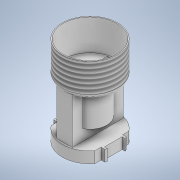
# Autodesk Inventor part: bulbholder
Saved by Autodesk Inventor 2020 (Build 240168000, 168)
## iProperties
Created: 2020-09-10
Part Number: bulbholder
Material: Generic
Document SubType Name: Modeling
Designer: zgoh017
Density: 1 g/cm^3
Appearance: Default
Author: zgoh017
Autodesk Inventor part; units mm, degrees
ref_plane "YZ Plane" through (0, 0, 0) normal (1, 0, 0) x (0, 1, 0)
ref_plane "XZ Plane" through (0, 0, 0) normal (0, 1, 0) x (-1, 0, 0)
ref_plane "XY Plane" through (0, 0, 0) normal (0, 0, 1) x (1, 0, 0)
sketch "Sketch1" plane through (0, 0, 0) normal (0, 1, 0) x (-1, 0, 0)
  circle A0 centre (0, 0) radius 12.5
  dimension "d0" = 25
  constraints: 1 centre point, 1 coincident
  measures "d0" diameter of A0
extrude "Extrusion1" add sketch "Sketch1" along normal blind 5
sketch "Sketch2" plane through (0, 5, 0) normal (0, 1, 0) x (1, 0, 0)
  circle A0 centre (0, 0) radius 12.5 projected
  line L0 (-12.5, 0) -> (-10.5, 0)
  line L1 (-10.5, 0) -> (-10.5, 4)
  line L2 (-10.5, 4) -> (-11.8427, 4)
  line L3 (-10.5, 0) -> (-10.5, -4)
  line L4 (-10.5, -4) -> (-11.8427, -4)
  line L5 (12.5, 0) -> (10.5, 0)
  line L6 (10.5, 0) -> (10.5, 4)
  line L7 (10.5, 4) -> (11.8427, 4)
  line L8 (10.5, 0) -> (10.5, -4)
  line L9 (10.5, -4) -> (11.8427, -4)
  dimension "d3" = 2
  dimension "d4" = 4
  dimension "d5" = 4
  dimension "d6" = 2
  dimension "d28" = 4
  dimension "d29" = 4
  constraints: 20 end point, 6 point on circle, 5 perpendicular, 3 horizontal, 2 point on line
  measures "d3" distance of L0.start L0.end
  measures "d4" distance of L0.end L1.end
  measures "d5" distance of L0.end L3.end
  measures "d6" distance of L5.start L5.end
  measures "d28" distance of L5.end L6.end
  measures "d29" distance of L5.end L8.end
extrude "Extrusion2" cut sketch "Sketch2" against normal through all contours L5 L6 L7 A0 | A0 L9 L8 L5 | L2 L1 L0 A0 | A0 L0 L3 L4
sketch "Sketch4" plane through (0, 5, 0) normal (0, 1, 0) x (1, 0, 0)
  line L0 (3.5, -11.5) -> (-3.5, -11.5)
  line L1 (-3.5, -11.5) -> (-3.5, 11.5)
  line L2 (-3.5, 11.5) -> (3.5, 11.5)
  line L3 (3.5, 11.5) -> (3.5, -11.5)
  line L4 (3.5, -11.5) -> (-3.5, 11.5) construction
  line L5 (-3.5, -11.5) -> (3.5, 11.5) construction
  point P0 (0, 0)
  dimension "d9" = 7
  dimension "d10" = 23
  constraints: 12 end point, 2 midpoint, 2 parallel, 1 horizontal, 1 perpendicular
  measures "d9" distance of L1.end L2.end
  measures "d10" distance of L0.end L1.end
extrude "Extrusion3" add sketch "Sketch4" along normal blind 5
sketch "Sketch5" plane through (0, 10, 0) normal (0, 1, 0) x (1, 0, 0)
  line L0 (-3.5, -11.5) -> (-3.5, 11.5) projected
  line L1 (-3.5, 6.6725) -> (-3.5, 11.5)
  line L2 (-3.5, 11.5) -> (3.5, 11.5) projected
  line L3 (-3.5, 11.5) -> (3.5, 11.5)
  line L4 (3.5, 11.5) -> (3.5, 6.6725)
  line L5 (3.5, 11.5) -> (3.5, -11.5) projected
  line L6 (-3.5, -6.6725) -> (-3.5, -11.5)
  line L7 (-3.5, -11.5) -> (3.5, -11.5)
  line L8 (3.5, -11.5) -> (3.5, -6.6725)
  arc A0 (3.5, -6.6725) -> (3.5, 6.6725) centre (0, 0) ccw
  arc A1 (-3.5, 6.6725) -> (-3.5, -6.6725) centre (0, 0) ccw
  constraints: 12 end point, 5 point on line, 4 point on circle, 2 centre point, 2 collinear, 1 coincident, 1 perpendicular, 1 vertical
extrude "Extrusion4" add sketch "Sketch5" along normal blind 15
sketch "Sketch6" plane through (0, 25, 0) normal (0, 1, 0) x (1, 0, 0)
  line L0 (-3.5, 11.5) -> (3.5, 11.5) projected
  line L1 (3.5, 11.5) -> (3.5, 6.6725) projected
  arc A0 (3.5, -6.6725) -> (3.5, 6.6725) centre (0, 0) ccw projected
  line L2 (3.5, -6.6725) -> (3.5, -11.5) projected
  line L3 (3.5, -11.5) -> (-3.5, -11.5) projected
  line L4 (-3.5, -11.5) -> (-3.5, -6.6725) projected
  arc A1 (-3.5, 6.6725) -> (-3.5, -6.6725) centre (0, 0) ccw projected
  line L5 (-3.5, 6.6725) -> (-3.5, 11.5) projected
  line L6 (-3.2721, -6.5332) -> (-3.2721, -11.2721)
  line L7 (-3.2721, -11.2721) -> (3.2721, -11.2721)
  line L8 (3.2721, -11.2721) -> (3.2721, -6.5332)
  arc A2 (3.2721, -6.5332) -> (3.2721, 6.5332) centre (0, 0) ccw
  line L9 (3.2721, 6.5332) -> (3.2721, 11.2721)
  line L10 (3.2721, 11.2721) -> (-3.2721, 11.2721)
  line L11 (-3.2721, 11.2721) -> (-3.2721, 6.5332)
  arc A3 (-3.2721, 6.5332) -> (-3.2721, -6.5332) centre (0, 0) ccw
  constraints: 12 end point, 4 point on circle, 2 centre point, 7 other
extrude "Extrusion5" cut sketch "Sketch6" against normal mid plane 14.5 contours A3 L11 L10 L9 A2 L8 L7 L6
sketch "Sketch7" plane through (0, 25, 0) normal (0, 1, 0) x (1, 0, 0)
  circle A0 centre (0, 0) radius 12.5
  constraints: 1 centre point, 1 coincident
extrude "Extrusion6" add sketch "Sketch7" along normal blind 15
sketch "Sketch8" plane through (0, 40, 0) normal (0, 1, 0) x (1, 0, 0)
  circle A0 centre (0, 0) radius 12.5 projected
  circle A1 centre (0, 0) radius 12.083
  constraints: 1 centre point
extrude "Extrusion7" cut sketch "Sketch8" against normal blind 14 contours A1
fillet "Fillet1" radius 2 1 edges at (-12.5, 25, 0)
sketch "Sketch9" plane through (0, 26, 0) normal (0, 1, 0) x (1, 0, 0)
  line L0 (-3.2721, -6.5332) -> (-3.2721, -11.2721)
  line L1 (-3.2721, -11.2721) -> (3.2721, -11.2721)
  line L2 (3.2721, -11.2721) -> (3.2721, -6.5332)
  arc A0 (3.2721, -6.5332) -> (3.2721, 6.5332) centre (0, 0) ccw
  line L3 (3.2721, 6.5332) -> (3.2721, 11.2721)
  line L4 (3.2721, 11.2721) -> (-3.2721, 11.2721)
  line L5 (-3.2721, 11.2721) -> (-3.2721, 6.5332)
  arc A1 (-3.2721, 6.5332) -> (-3.2721, -6.5332) centre (0, 0) ccw
  constraints: 12 end point, 4 point on circle, 2 centre point
extrude "Extrusion8" cut sketch "Sketch9" against normal blind 15.5
thread "Thread1" size "M25x2" class "6g" standard "ANSI Metric M Profile" full length
thread "Thread2" size "M15x1.5" class "6H" standard "ANSI Metric M Profile" full length
sketch "Sketch10" plane through (-3.5, 5, 11.5) normal (0, 0, 1) x (1, 0, 0)
  point P0 (3.5, -5)
sketch "Sketch11" plane through (0, 5, 0) normal (0, 1, 0) x (1, 0, 0)
  arc A0 (-11.8427, -4) -> (11.8427, -4) centre (0, 0) ccw projected
  line L0 (-11.5197, -4.8526) -> (-9.8427, -4.8526)
  line L1 (-9.8427, -4.8526) -> (-9.8427, -7.7052)
  arc A1 (11.8427, 4) -> (-11.8427, 4) centre (0, 0) ccw projected
  line L2 (11.5197, -4.8526) -> (9.8427, -4.8526)
  line L3 (9.8427, -4.8526) -> (9.8427, -7.7052)
  line L4 (-10.5, -4) -> (-10.5, 4) projected
  line L5 (10.5, 4) -> (10.5, -4) projected
  line L6 (-11.5197, 4.8526) -> (-9.8427, 4.8526)
  line L7 (-9.8427, 4.8526) -> (-9.8427, 7.7052)
  line L8 (11.5197, 4.8526) -> (9.8427, 4.8526)
  line L9 (9.8427, 4.8526) -> (9.8427, 7.7052)
  constraints: 16 end point, 2 point on circle, 1 horizontal, 1 perpendicular
extrude "Extrusion9" cut sketch "Sketch11" against normal through all
body "Solid1"
